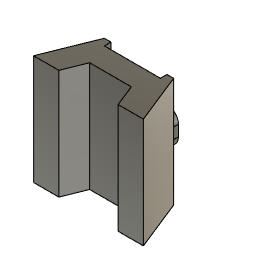
ClimbSim_Slide v2 (Autodesk Fusion 360 design; units mm, degrees)
Autodesk Fusion 360 part; units mm, degrees
sketch "スケッチ2" plane through (0, 0, 0) normal (0, 0, 1) x (1, 0, 0)
  line L0 (15.8, 3) -> (25, -20)
  line L1 (-25, -20) -> (-15.8, 3)
  line L2 (-13.5, -20) -> (-9.5, -10)
  line L3 (-9.5, -10) -> (9.5, -10)
  line L4 (9.5, -10) -> (13.5, -20)
  line L5 (13.5, -20) -> (25, -20)
  line L6 (-13.5, -20) -> (-25, -20)
  line L7 (-15.8, 3) -> (-12.75, 3)
  line L8 (-12.75, 3) -> (-12.75, 0)
  line L9 (-12.75, 0) -> (12.75, 0)
  line L10 (12.75, 0) -> (12.75, 3)
  line L11 (12.75, 3) -> (15.8, 3)
  dimension "d1" = 19
  dimension "d2" = 9.5
  dimension "d5" = 13
  dimension "d6" = 10
  dimension "d7" = 25.5
  dimension "d8" = 3
  dimension "d9" = 11.5
  dimension "d24" = 25
  dimension "d25" = 12.75
  dimension "d26" = 20
  constraint horizontal L6
  constraint horizontal L5
  constraint equal L5 L6
  constraint horizontal L2.start L4.end
  constraint perpendicular L7 L8
  constraint perpendicular L8 L9
  constraint perpendicular L9 L10
  constraint equal L7 L11
  constraint horizontal L3
  constraint horizontal origin L8.end
  constraint equal L0 L1
  constraint parallel L1 L2
  constraint horizontal L9
  constraint horizontal L11
  measures "d1" distance of L2.end L3.end
  measures "d2" horizontal distance of origin L2.end
  measures "d5" vertical distance of L1.end L2.end
  measures "d6" vertical distance of L3.end L4.end
  measures "d7" distance of L8.end L9.end
  measures "d8" distance of L9.end L10.end
  measures "d9" distance of L0.end L4.end
  measures "d24" horizontal distance of origin L1.start
  measures "d25" horizontal distance of origin L7.end
  measures "d26" vertical distance of origin L1.start
extrude "押し出し1" add sketch "スケッチ2" along normal blind 50
sketch "スケッチ3" plane through (0, 0, 0) normal (0, 1, 0) x (1, 0, 0)
  line L0 (5, -20) -> (5, -15)
  arc A0 (5, -15) -> (-5, -15) centre (0, -15) ccw
  line L1 (-5, -15) -> (-5, -20)
  arc A1 (-5, -20) -> (5, -20) centre (0, -20) ccw
  line L2 (0, -20) -> (0, -15) construction
  dimension "d16" = 5
  dimension "d17" = 5
  constraint tangent L0 A0
  constraint tangent A0 L1
  constraint parallel L0 L1
  constraint tangent L1 A1
  constraint tangent L0 A1
  constraint vertical L2
  measures "d16" radius of A0
  measures "d17" distance of L0.start L0.end
extrude "押し出し2" add sketch "スケッチ3" along normal blind 16
sketch "スケッチ6" plane through (0, 0, 0) normal (1, 0, 0) x (0, 1, 0)
  circle A0 centre (10, 17.5) radius 3
  line L0 (0, 0) -> (0, 50)
  dimension "d21" = 6
  dimension "d22" = 10
  measures "d21" diameter of A0
  measures "d22" distance of A0.centre L0
extrude "押し出し4" cut sketch "スケッチ6" along normal through all and the other way through all
